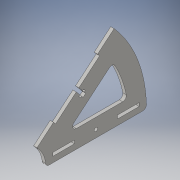
# Autodesk Inventor part: SideMount
Saved by Autodesk Inventor 2016 (Build 200138000, 138)
## iProperties
Created: 2016-07-10
Part Number: SideMount
Material: Generic
Document SubType Name: Modeling
Designer: jeffkub
Density: 1 g/cm^3
Appearance: Default
Author: jeffkub
Autodesk Inventor part; units mm, degrees
ref_plane "YZ Plane" through (0, 0, 0) normal (1, 0, 0) x (0, 1, 0)
ref_plane "XZ Plane" through (0, 0, 0) normal (0, 1, 0) x (-1, 0, 0)
ref_plane "XY Plane" through (0, 0, 0) normal (0, 0, 1) x (1, 0, 0)
sketch "Sketch1" plane through (0, 0, 0) normal (1, 0, 0) x (0, 1, 0)
  line L0 (18.4717, 7.7423) -> (30.7168, -6.8509)
  line L1 (75.6155, -60.3591) -> (73.4706, -62.1589)
  line L2 (73.4706, -62.1589) -> (61.2255, -47.5657) construction
  line L3 (16.3268, 5.9425) -> (18.4717, 7.7423)
  line L4 (30.7168, -6.8509) -> (28.5719, -8.6507)
  line L5 (63.3704, -45.7659) -> (61.2255, -47.5657)
  line L6 (30.7168, -6.8509) -> (63.3704, -45.7659) construction
  line L7 (63.3704, -45.7659) -> (75.6155, -60.3591)
  line L8 (61.2255, -47.5657) -> (45.895, -29.2956)
  line L9 (28.5719, -8.6507) -> (16.3268, 5.9425) construction
  arc A0 (2.8222, 0.1573) -> (16.3268, 5.9425) centre (0, 25.4) ccw
  line L10 (0, -2.9981) -> (0, -85.6796)
  arc A1 (3.2657, -88.8533) -> (73.4706, -62.1589) centre (0, 25.4) ccw
  arc A2 (2.8222, 0.1573) -> (0, -2.9981) centre (3.175, -2.9981) ccw
  arc A3 (0, -85.6796) -> (3.2657, -88.8533) centre (3.175, -85.6796) ccw
  line L11 (5, -6.2388) -> (8, -6.2388)
  line L12 (8, -6.2388) -> (8, -25.2888)
  line L13 (8, -82.4388) -> (5, -82.4388)
  line L14 (5, -82.4388) -> (5, -63.3888)
  line L15 (8, -25.2888) -> (5, -25.2888)
  line L16 (8, -63.3888) -> (5, -63.3888)
  line L17 (8, -25.2888) -> (8, -63.3888) construction
  line L18 (5, -25.2888) -> (5, -6.2388)
  line L19 (5, -63.3888) -> (5, -25.2888) construction
  line L20 (8, -63.3888) -> (8, -82.4388)
  circle A4 centre (6.5, -44.3388) radius 1.5
  line L21 (51.7389, -22.3686) -> (29.8853, -40.706)
  line L22 (43.9024, -26.9208) -> (40.0722, -30.1348)
  line L23 (40.0722, -30.1348) -> (39.6966, -29.6872)
  line L24 (39.333, -29.2538) -> (38.8996, -29.6174) construction
  line L25 (37.4945, -30.7965) -> (38.2337, -31.6775)
  line L26 (38.2337, -31.6775) -> (36.7016, -32.963)
  line L27 (36.7016, -32.963) -> (37.6979, -34.1504)
  arc A5 (39.6966, -29.6872) -> (39.333, -29.2538) centre (39.2981, -29.6523) ccw
  line L28 (39.6966, -29.6872) -> (39.333, -29.2538) construction
  line L29 (38.8996, -29.6174) -> (37.4945, -30.7965)
  arc A6 (39.333, -29.2538) -> (38.8996, -29.6174) centre (39.2981, -29.6523) ccw
  line L30 (45.895, -29.2956) -> (42.0648, -32.5095)
  line L31 (42.0648, -32.5095) -> (42.4404, -32.9571)
  line L32 (40.9655, -34.9332) -> (40.2263, -34.0522)
  line L33 (40.2263, -34.0522) -> (38.6942, -35.3378)
  line L34 (38.6942, -35.3378) -> (37.6979, -34.1504)
  arc A7 (42.804, -33.3905) -> (42.4404, -32.9571) centre (42.4055, -33.3556) ccw
  line L35 (42.3707, -33.7541) -> (40.9655, -34.9332)
  arc A8 (42.3707, -33.7541) -> (42.804, -33.3905) centre (42.4055, -33.3556) ccw
  line L36 (43.9024, -26.9208) -> (28.5719, -8.6507)
  line L37 (45.895, -29.2956) -> (43.9024, -26.9208)
  line L38 (15.875, -26.9394) -> (15.875, -67.9256)
  line L39 (21.4822, -24.8986) -> (47.8276, -56.2958)
  arc A9 (19.685, -71.0364) -> (46.9085, -61.1279) centre (0, 25.4) ccw
  arc A10 (21.4822, -24.8986) -> (15.875, -26.9394) centre (19.05, -26.9394) ccw
  arc A11 (15.875, -67.9256) -> (19.685, -71.0364) centre (19.05, -67.9256) ccw
  arc A12 (46.9085, -61.1279) -> (47.8276, -56.2958) centre (45.3954, -58.3366) ccw
  point P0 (0, 0)
  point P1 (0, 0)
  point P2 (0, -88.9)
  point P3 (75.5935, -60.3328)
  point P4 (0, -44.3388)
  point P5 (5, -44.3388)
  point P6 (6.5, -25.2888)
  point P7 (44.8987, -28.1082)
  point P8 (15.875, -71.7363)
  point P9 (50.2771, -59.215)
  point P10 (15.875, -71.7363)
  dimension "d0" = 2.8
  dimension "d1" = 88.9
  dimension "d2" = 19.05
  dimension "d3" = 19.05
  dimension "d4" = 40
  dimension "d5" = 25.4
  dimension "d6" = 3.175
  dimension "d7" = 3
  dimension "d8" = 76.2
  dimension "d9" = 5
  dimension "d10" = 19.05
  dimension "d11" = 3
  dimension "d12" = 3.1
  dimension "d13" = 5.4
  dimension "d14" = 5
  dimension "d15" = 0.4
  dimension "d16" = 2.4
  dimension "d17" = 2
  dimension "d22" = 15.875
  dimension "d23" = 15.875
  dimension "d24" = 15.875
  dimension "d25" = 3.175
  constraints: 80 end point, 31 perpendicular, 29 point on circle, 28 parallel, 15 point on line, 13 centre point, 12 tangent, 9 symmetric about line, 3 equal length, 3 equal radius, 3 midpoint, 2 coincident, 2 horizontal alignment, 2 line through centre, 2 vertical, 1 horizontal, 1 vertical alignment, 2 other
  measures "d0" distance of L1.end L1.start
  measures "d1" distance of L0.start L1.start
  measures "d2" distance of L5.start L1.start
  measures "d3" distance of L0.start L0.end
  measures "d4" angle of L10 L8
  measures "d5" radius of A0
  measures "d6" radius of A2
  measures "d7" distance of L13.start L13.end
  measures "d8" distance between parallel lines of L13 L11
  measures "d9" distance between parallel lines of L10 L19
  measures "d10" distance of L11.end L12.end
  measures "d11" diameter of A4
  measures "d12" diameter of L22 L21
  measures "d13" diameter of L24 L21
  measures "d14" distance between parallel lines of L23 L8
  measures "d15" radius of A6
  measures "d16" distance between parallel lines of L25 L23
  measures "d17" distance of L25.end L26.end
  measures "d22" distance between parallel lines of L36 L39
  measures "d23" distance between parallel lines of L10 L38
  measures "d24" radial gap between concentric circles of A1 A9
  measures "d25" radius of A10
extrude "Extrusion1" add sketch "Sketch1" along normal blind 3 contours L0 L4 L36 L22 L23 A5 A6 L29 L25 L26 L27 L34 L33 L32 L35 A8 A7 L31 L30 L8 L5 L7 L1 A1 A3 L10 A2 A0 L3
equation "\"d3\" = d2"
equation "\"d23\" = d22"
equation "\"d24\" = d22"
body "Solid1"
